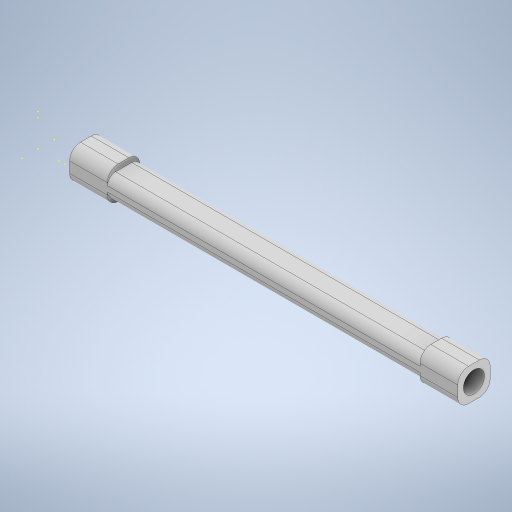
# Autodesk Inventor part: Part4
Saved by Autodesk Inventor 2024 (Build 280153000, 153)
## iProperties
Created: 2023-10-06
Part Number: Part4
Material: Generic
Document SubType Name: Modeling
Designer: kubad
Density: 1 g/cm^3
Appearance: Default
Author: kubad
## iProperties of the stored document Part3_3DPrint.ipt
Created: 2023-10-06
Part Number: Part3_3DPrint
Material: Generic
Document SubType Name: Modeling
Designer: kubad
Density: 1 g/cm^3
Appearance: Default
Author: kubad
Autodesk Inventor part; units mm, degrees
ref_plane "YZ Plane" through (0, 0, 0) normal (1, 0, 0) x (0, 1, 0)
ref_plane "XZ Plane" through (0, 0, 0) normal (0, 1, 0) x (-1, 0, 0)
ref_plane "XY Plane" through (0, 0, 0) normal (0, 0, 1) x (1, 0, 0)
sketch "Sketch1" plane through (0, 0, 0) normal (0, 1, 0) x (-1, 0, 0)
  point P0 (0, 0)
sketch "Sketch2" plane through (0, 0, 0) normal (0, 1, 0) x (-1, 0, 0)
  circle A0 centre (0, 0) radius 3.85
  dimension "d0" = 7.7
  constraints: 1 centre point, 1 coincident
  measures "d0" diameter of A0
extrude "Extrusion1" add sketch "Sketch2" along normal blind 6
sketch "Sketch3" plane through (0, 6, 0) normal (0, 1, 0) x (1, 0, 0)
  circle A0 centre (0, 0) radius 1
  dimension "d3" = 2
  constraints: 1 centre point, 1 coincident
  measures "d3" diameter of A0
extrude "Extrusion2" cut sketch "Sketch3" against normal through all
sketch "Sketch4" plane through (0, 0, 0) normal (0, -1, 0) x (1, 0, 0)
  circle A0 centre (0, 0) radius 3.85 projected
  line L0 (0, 3.85) -> (3.85, 3.85)
  line L1 (3.85, 3.85) -> (3.85, -3.85)
  line L2 (3.85, -3.85) -> (0, -3.85)
  line L3 (3.85, 3.85) -> (4.85, 3.85)
  line L4 (4.85, 3.85) -> (4.85, -3.85)
  line L5 (4.85, -3.85) -> (3.85, -3.85)
  line L6 (3.85, -3.85) -> (3.85, 3.85)
  line L7 (4.85, 3.85) -> (4.85, 3)
  line L8 (4.85, -3.85) -> (4.85, -3)
  line L9 (4.85, 3) -> (3.85, 3)
  line L10 (3.85, 3) -> (3.85, -3)
  line L11 (3.85, -3) -> (4.85, -3)
  line L12 (4.85, -3) -> (4.85, 3)
  point P0 (3.85, -3)
  dimension "d6" = 1
  dimension "d7" = 0.85
  dimension "d8" = 0.85
  constraints: 26 end point, 5 parallel, 4 point on line, 3 horizontal, 3 perpendicular, 1 vertical alignment, 1 other
  measures "d6" distance of L4.end L5.end
  measures "d7" distance of L3.end L7.end
  measures "d8" distance of L4.end L8.end
extrude "Extrusion3" add sketch "Sketch4" against normal blind 6 contours L1 L9 L4 L11
sketch "Sketch5" plane through (4.85, 0, 3) normal (1, 0, 0) x (0, 0, -1)
  line L0 (6.85, 0) -> (-0.85, 0) projected
  line L1 (6, 0) -> (6, 6) projected
  line L2 (0.0003, 0) -> (6, 0)
  line L3 (6, 0) -> (6, 1)
  line L4 (6, 1) -> (0.0003, 1)
  line L5 (0.0003, 1) -> (0.0003, 0)
  line L6 (6.85, 6) -> (-0.85, 6) projected
  line L7 (0.0003, 6) -> (6, 6)
  line L8 (6, 6) -> (6, 5)
  line L9 (6, 5) -> (0.0003, 5)
  line L10 (0.0003, 5) -> (0.0003, 6)
  point P0 (3, 0)
  point P1 (3, 6)
  dimension "d11" = 1
  dimension "d12" = 1
  constraints: 16 end point, 4 parallel, 4 point on line, 2 horizontal, 2 perpendicular
  measures "d11" distance of L3.end L2.end
  measures "d12" distance of L7.end L8.end
extrude "Extrusion4" cut sketch "Sketch5" against normal blind 1 contours L9 L10 L6 L1
extrude "Extrusion5" cut sketch "Sketch5" against normal blind 1 contours L0 L5 L4 L1
sketch "Sketch6" plane through (4.85, 5, 2.9997) normal (0, 0, -1) x (-1, 0, 0)
  line L0 (0, 0) -> (1, 0) projected
  line L1 (0, -5) -> (0, 1) projected
  line L2 (1, 0) -> (0, 0)
  line L3 (0, 0) -> (0, 1)
  line L4 (0, 1) -> (1, 1)
  line L5 (1, 1) -> (1, 0)
  line L6 (1, -5) -> (0, -5)
  line L7 (0, -5) -> (0, -3.9916)
  line L8 (0, -3.9916) -> (1, -3.9916)
  line L9 (1, -3.9916) -> (1, -5)
  point P0 (4.85, -5)
  constraints: 16 end point, 4 parallel, 2 horizontal, 2 perpendicular, 2 point on line
extrude "Extrusion6" cut sketch "Sketch6" against normal through all contours L1 L4 L5 L0
extrude "Extrusion7" cut sketch "Sketch6" against normal through all contours L1 L8 L9 L6
sketch "Sketch7" plane through (4.85, 5, 3) normal (1, 0, 0) x (0, 0, -1)
  line L0 (0, 0) -> (3, 0) projected
  line L1 (6, -4) -> (6, 0) projected
  line L2 (0, 0) -> (6, 0)
  line L3 (6, 0) -> (6, -4)
  line L4 (6, -4) -> (0, -4)
  line L5 (0, -4) -> (0, 0)
  point P0 (3, -5)
  constraints: 8 end point, 2 parallel, 1 horizontal, 1 perpendicular
extrude "Extrusion8" add sketch "Sketch7" along normal blind 71
sketch "Sketch8" plane through (3.85, 1, -3) normal (0, 0, -1) x (-1, 0, 0)
  point P0 (3.85, -1)
sketch "Sketch9" plane through (3.85, 5, 0) normal (0, 1, 0) x (1, 0, 0)
  line L0 (72, 3) -> (72, -3) projected
  line L1 (72, 0) -> (75.85, 0)
  circle A0 centre (75.85, 0) radius 3.85
  point P0 (-3.85, 0)
  dimension "d23" = 3.85
  constraints: 2 end point, 1 coincident, 1 horizontal, 1 horizontal alignment, 1 midpoint, 2 other
  measures "d23" distance of L1.start L1.end
extrude "Extrusion9" add sketch "Sketch9" along normal blind 1
extrude "Extrusion10" add sketch "Sketch9" against normal blind 5
sketch "Sketch10" plane through (79.7, 6, 0) normal (0, 1, 0) x (1, 0, 0)
  circle A0 centre (0, 0) radius 1.85
  point P0 (-79.7, 0)
  dimension "d28" = 3.7
  constraints: 1 centre point
  measures "d28" diameter of A0
extrude "Extrusion11" cut sketch "Sketch10" against normal through all
sketch "Sketch11" plane through (3.85, 5, 0) normal (-1, 0, 0) x (0, 0, 1)
  point P0 (0, -5)
sketch "Sketch12" plane through (3.85, 5, -3) normal (-1, 0, 0) x (0, 0, 1)
  line L0 (0, 0) -> (3, 0) projected
  line L1 (6, 0) -> (6, -4) projected
  line L2 (0, 0) -> (6, 0)
  line L3 (6, 0) -> (6, -4)
  line L4 (6, -4) -> (0, -4)
  line L5 (0, -4) -> (0, 0)
  point P0 (3, -5)
  constraints: 8 end point, 2 parallel, 1 horizontal, 1 perpendicular
extrude "Extrusion12" add sketch "Sketch12" along normal blind 2
sketch "Sketch13" plane through (75.85, 5, 3) normal (1, 0, 0) x (0, 0, -1)
  line L0 (3, 0) -> (0, 0) projected
  line L1 (3, -4) -> (6, -4) projected
  line L2 (0, 0) -> (6, 0)
  line L3 (6, 0) -> (6, -4)
  line L4 (6, -4) -> (0, -4)
  line L5 (0, -4) -> (0, 0)
  point P0 (3, -5)
  constraints: 8 end point, 2 parallel, 1 horizontal, 1 perpendicular
extrude "Extrusion13" add sketch "Sketch13" along normal blind 1.6
fillet "Fillet1" radius 1.5 1 edges at (39.85, 5, 3)
fillet "Fillet2" radius 1.5 1 edges at (39.85, 5, -3)
fillet "Fillet3" radius 1.5 1 edges at (39.85, 1, -3)
fillet "Fillet4" radius 1.5 1 edges at (41.0685, 1, 3)
sketch "Sketch14" plane through (3.5458, 5, 1.5) normal (0, 1, 0) x (1, 0, 0)
  point P0 (-3.5458, 1.5)
sketch "Sketch15" plane through (3.5458, 5, 1.5) normal (0, 1, 0) x (1, 0, 0)
  line L0 (0.4177, 2.9988) -> (2.9717, 2.9988) construction
  line L1 (2.9717, 2.9988) -> (2.9717, -0.0492) construction
  line L2 (2.9717, -0.0492) -> (0.4177, -0.0492) construction
  line L3 (0.4177, -0.0492) -> (0.4177, 2.9988) construction
  line L4 (0.398, -0.0492) -> (1.4255, 2.9988)
  line L5 (1.4255, 2.9988) -> (1.9244, 2.9988)
  line L6 (1.9244, 2.9988) -> (2.952, -0.0492)
  line L7 (2.952, -0.0492) -> (2.5247, -0.0492)
  line L8 (2.5247, -0.0492) -> (2.248, 0.803)
  line L9 (2.248, 0.803) -> (1.0846, 0.803)
  line L10 (1.0846, 0.803) -> (0.808, -0.0492)
  line L11 (0.808, -0.0492) -> (0.398, -0.0492)
  line L12 (2.1369, 1.1488) -> (1.6651, 2.5839)
  line L13 (1.6651, 2.5839) -> (1.1958, 1.1488)
  line L14 (1.1958, 1.1488) -> (2.1369, 1.1488)
  point P0 (-3.5458, 1.5)
  constraints: 2 other
extrude "Extrusion14" add sketch "Sketch15" along normal blind 0.2
sketch "Sketch16" plane through (3.5458, 5, -1.5) normal (0, 1, 0) x (1, 0, 0)
  line L0 (69.8363, -0.0038) -> (72.3064, -0.0038) construction
  line L1 (72.3064, -0.0038) -> (72.3064, -3.0518) construction
  line L2 (72.3064, -3.0518) -> (69.8363, -3.0518) construction
  line L3 (69.8363, -3.0518) -> (69.8363, -0.0038) construction
  spline S0 degree 2 poles (72.2125, -2.1157) (72.2125, -2.3429) (72.0396, -2.6912) (71.8963, -2.8048) knots 0 0 0 1 2 2 2
  spline S1 degree 2 poles (71.8963, -2.8048) (71.7234, -2.9382) (71.3307, -3.0518) (71.0195, -3.0518) knots 0 0 0 1 2 2 2
  line L4 (71.0195, -3.0518) -> (70.1451, -3.0518)
  line L5 (70.1451, -3.0518) -> (70.1451, -0.0038)
  line L6 (70.1451, -0.0038) -> (70.9528, -0.0038)
  spline S2 degree 2 poles (70.9528, -0.0038) (71.2788, -0.0038) (71.6049, -0.0458) (71.7531, -0.1273) knots 0 0 0 1 2 2 2
  spline S3 degree 2 poles (71.7531, -0.1273) (71.9186, -0.2138) (72.0692, -0.4978) (72.0692, -0.6905) knots 0 0 0 1 2 2 2
  spline S4 degree 2 poles (72.0692, -0.6905) (72.0692, -0.9054) (71.842, -1.2462) (71.6419, -1.3426) knots 0 0 0 1 2 2 2
  line L7 (71.6419, -1.3426) -> (71.6419, -1.3574)
  spline S5 degree 2 poles (71.6419, -1.3574) (71.9136, -1.4315) (72.2125, -1.8242) (72.2125, -2.1157) knots 0 0 0 1 2 2 2
  spline S6 degree 2 poles (71.7901, -2.133) (71.7901, -1.9601) (71.6913, -1.7378) (71.5431, -1.6587) knots 0 0 0 1 2 2 2
  spline S7 degree 2 poles (71.5431, -1.6587) (71.4468, -1.6093) (71.2195, -1.5797) (71.0096, -1.5797) knots 0 0 0 1 2 2 2
  line L8 (71.0096, -1.5797) -> (70.5502, -1.5797)
  line L9 (70.5502, -1.5797) -> (70.5502, -2.706)
  line L10 (70.5502, -2.706) -> (70.8787, -2.706)
  spline S8 degree 2 poles (70.8787, -2.706) (71.1454, -2.706) (71.4517, -2.6566) (71.5703, -2.5776) knots 0 0 0 1 2 2 2
  spline S9 degree 2 poles (71.5703, -2.5776) (71.6839, -2.4961) (71.7901, -2.2935) (71.7901, -2.133) knots 0 0 0 1 2 2 2
  spline S10 degree 2 poles (71.6469, -0.7473) (71.6469, -0.6386) (71.5728, -0.4756) (71.4912, -0.4287) knots 0 0 0 1 2 2 2
  spline S11 degree 2 poles (71.4912, -0.4287) (71.3924, -0.3743) (71.1529, -0.3496) (70.938, -0.3496) knots 0 0 0 1 2 2 2
  line L11 (70.938, -0.3496) -> (70.5502, -0.3496)
  line L12 (70.5502, -0.3496) -> (70.5502, -1.2413)
  line L13 (70.5502, -1.2413) -> (71.0096, -1.2413)
  spline S12 degree 2 poles (71.0096, -1.2413) (71.1998, -1.2413) (71.3801, -1.2018) (71.4764, -1.14) knots 0 0 0 1 2 2 2
  spline S13 degree 2 poles (71.4764, -1.14) (71.5703, -1.0807) (71.6469, -0.8905) (71.6469, -0.7473) knots 0 0 0 1 2 2 2
  point P0 (-3.5458, -1.5)
  constraints: 2 other
extrude "Extrusion15" add sketch "Sketch16" along normal blind 0.2
sketch "Sketch17" plane through (3.5458, 5, -1.5) normal (0, 1, 0) x (1, 0, 0)
  line L0 (0.4145, -1.5) -> (36.4145, -1.5)
  line L1 (30.4487, 0.0859) -> (55.6072, 0.0859) construction
  line L2 (55.6072, 0.0859) -> (55.6072, -2.5363) construction
  line L3 (55.6072, -2.5363) -> (30.4487, -2.5363) construction
  line L4 (30.4487, -2.5363) -> (30.4487, 0.0859) construction
  line L5 (32.5853, -0.4353) -> (31.2663, -3.0264)
  line L6 (31.2663, -3.0264) -> (30.8316, -3.0264)
  line L7 (30.8316, -3.0264) -> (32.2247, -0.3365)
  line L8 (32.2247, -0.3365) -> (30.6513, -0.3365)
  line L9 (30.6513, -0.3365) -> (30.6513, 0.0216)
  line L10 (30.6513, 0.0216) -> (32.5853, 0.0216)
  line L11 (32.5853, 0.0216) -> (32.5853, -0.4353)
  line L12 (34.838, -3.0264) -> (32.9583, -3.0264)
  line L13 (32.9583, -3.0264) -> (32.9583, -2.5941)
  spline S0 degree 2 poles (32.9583, -2.5941) (33.1608, -2.4039) (33.5214, -2.0507) (33.6943, -1.8605) knots 0 0 0 1 2 2 2
  spline S1 degree 2 poles (33.6943, -1.8605) (34.0426, -1.4777) (34.297, -1.0182) (34.297, -0.7737) knots 0 0 0 1 2 2 2
  spline S2 degree 2 poles (34.297, -0.7737) (34.297, -0.6453) (34.218, -0.4526) (34.1464, -0.3909) knots 0 0 0 1 2 2 2
  spline S3 degree 2 poles (34.1464, -0.3909) (34.0747, -0.3291) (33.887, -0.2674) (33.7734, -0.2674) knots 0 0 0 1 2 2 2
  spline S4 degree 2 poles (33.7734, -0.2674) (33.6647, -0.2674) (33.4424, -0.3217) (33.3411, -0.3637) knots 0 0 0 1 2 2 2
  spline S5 degree 2 poles (33.3411, -0.3637) (33.2547, -0.3983) (33.0941, -0.4971) (33.0447, -0.5317) knots 0 0 0 1 2 2 2
  line L14 (33.0447, -0.5317) -> (33.0225, -0.5317)
  line L15 (33.0225, -0.5317) -> (33.0225, -0.0969)
  spline S6 degree 2 poles (33.0225, -0.0969) (33.1485, -0.0352) (33.6005, 0.0859) (33.803, 0.0859) knots 0 0 0 1 2 2 2
  spline S7 degree 2 poles (33.803, 0.0859) (34.2303, 0.0859) (34.712, -0.3662) (34.712, -0.7515) knots 0 0 0 1 2 2 2
  spline S8 degree 2 poles (34.712, -0.7515) (34.712, -0.9318) (34.628, -1.2331) (34.5539, -1.3616) knots 0 0 0 1 2 2 2
  spline S9 degree 2 poles (34.5539, -1.3616) (34.4798, -1.495) (34.2649, -1.7568) (34.1464, -1.8828) knots 0 0 0 1 2 2 2
  spline S10 degree 2 poles (34.1464, -1.8828) (33.9537, -2.0927) (33.4819, -2.5422) (33.3411, -2.6732) knots 0 0 0 1 2 2 2
  line L16 (33.3411, -2.6732) -> (34.838, -2.6732)
  line L17 (34.838, -2.6732) -> (34.838, -3.0264)
  line L18 (37.8958, -3.0264) -> (37.8958, -1.7024)
  spline S11 degree 2 poles (37.8958, -1.7024) (37.8958, -1.5444) (37.8711, -1.2751) (37.8316, -1.201) knots 0 0 0 1 2 2 2
  spline S12 degree 2 poles (37.8316, -1.201) (37.7921, -1.1195) (37.6414, -1.0405) (37.5105, -1.0405) knots 0 0 0 1 2 2 2
  spline S13 degree 2 poles (37.5105, -1.0405) (37.392, -1.0405) (37.1203, -1.1862) (36.977, -1.3245) knots 0 0 0 1 2 2 2
  spline S14 degree 2 poles (36.977, -1.3245) (36.9795, -1.3591) (36.9844, -1.4554) (36.9844, -1.5197) knots 0 0 0 1 2 2 2
  line L19 (36.9844, -1.5197) -> (36.9844, -3.0264)
  line L20 (36.9844, -3.0264) -> (36.5991, -3.0264)
  line L21 (36.5991, -3.0264) -> (36.5991, -1.7024)
  spline S15 degree 2 poles (36.5991, -1.7024) (36.5991, -1.5444) (36.5744, -1.2751) (36.5349, -1.201) knots 0 0 0 1 2 2 2
  spline S16 degree 2 poles (36.5349, -1.201) (36.4953, -1.1195) (36.3447, -1.0405) (36.2138, -1.0405) knots 0 0 0 1 2 2 2
  spline S17 degree 2 poles (36.2138, -1.0405) (36.0903, -1.0405) (35.8161, -1.1961) (35.6876, -1.3171) knots 0 0 0 1 2 2 2
  line L22 (35.6876, -1.3171) -> (35.6876, -3.0264)
  line L23 (35.6876, -3.0264) -> (35.3023, -3.0264)
  line L24 (35.3023, -3.0264) -> (35.3023, -0.7391)
  line L25 (35.3023, -0.7391) -> (35.6876, -0.7391)
  line L26 (35.6876, -0.7391) -> (35.6876, -0.9911)
  spline S18 degree 2 poles (35.6876, -0.9911) (35.8383, -0.8404) (36.1347, -0.6749) (36.3126, -0.6749) knots 0 0 0 1 2 2 2
  spline S19 degree 2 poles (36.3126, -0.6749) (36.5151, -0.6749) (36.8288, -0.8602) (36.9103, -1.0701) knots 0 0 0 1 2 2 2
  spline S20 degree 2 poles (36.9103, -1.0701) (37.0857, -0.875) (37.4167, -0.6749) (37.6093, -0.6749) knots 0 0 0 1 2 2 2
  spline S21 degree 2 poles (37.6093, -0.6749) (37.7575, -0.6749) (37.9996, -0.7663) (38.0885, -0.87) knots 0 0 0 1 2 2 2
  spline S22 degree 2 poles (38.0885, -0.87) (38.1799, -0.9738) (38.2812, -1.285) (38.2812, -1.5197) knots 0 0 0 1 2 2 2
  line L27 (38.2812, -1.5197) -> (38.2812, -3.0264)
  line L28 (38.2812, -3.0264) -> (37.8958, -3.0264)
  line L29 (41.4156, -3.0264) -> (41.4156, -1.7024)
  spline S23 degree 2 poles (41.4156, -1.7024) (41.4156, -1.5444) (41.3909, -1.2751) (41.3514, -1.201) knots 0 0 0 1 2 2 2
  spline S24 degree 2 poles (41.3514, -1.201) (41.3119, -1.1195) (41.1612, -1.0405) (41.0303, -1.0405) knots 0 0 0 1 2 2 2
  spline S25 degree 2 poles (41.0303, -1.0405) (40.9117, -1.0405) (40.64, -1.1862) (40.4968, -1.3245) knots 0 0 0 1 2 2 2
  spline S26 degree 2 poles (40.4968, -1.3245) (40.4992, -1.3591) (40.5042, -1.4554) (40.5042, -1.5197) knots 0 0 0 1 2 2 2
  line L30 (40.5042, -1.5197) -> (40.5042, -3.0264)
  line L31 (40.5042, -3.0264) -> (40.1189, -3.0264)
  line L32 (40.1189, -3.0264) -> (40.1189, -1.7024)
  spline S27 degree 2 poles (40.1189, -1.7024) (40.1189, -1.5444) (40.0942, -1.2751) (40.0546, -1.201) knots 0 0 0 1 2 2 2
  spline S28 degree 2 poles (40.0546, -1.201) (40.0151, -1.1195) (39.8644, -1.0405) (39.7335, -1.0405) knots 0 0 0 1 2 2 2
  spline S29 degree 2 poles (39.7335, -1.0405) (39.61, -1.0405) (39.3359, -1.1961) (39.2074, -1.3171) knots 0 0 0 1 2 2 2
  line L33 (39.2074, -1.3171) -> (39.2074, -3.0264)
  line L34 (39.2074, -3.0264) -> (38.8221, -3.0264)
  line L35 (38.8221, -3.0264) -> (38.8221, -0.7391)
  line L36 (38.8221, -0.7391) -> (39.2074, -0.7391)
  line L37 (39.2074, -0.7391) -> (39.2074, -0.9911)
  spline S30 degree 2 poles (39.2074, -0.9911) (39.3581, -0.8404) (39.6545, -0.6749) (39.8323, -0.6749) knots 0 0 0 1 2 2 2
  spline S31 degree 2 poles (39.8323, -0.6749) (40.0349, -0.6749) (40.3486, -0.8602) (40.4301, -1.0701) knots 0 0 0 1 2 2 2
  spline S32 degree 2 poles (40.4301, -1.0701) (40.6054, -0.875) (40.9364, -0.6749) (41.1291, -0.6749) knots 0 0 0 1 2 2 2
  spline S33 degree 2 poles (41.1291, -0.6749) (41.2773, -0.6749) (41.5194, -0.7663) (41.6083, -0.87) knots 0 0 0 1 2 2 2
  spline S34 degree 2 poles (41.6083, -0.87) (41.6997, -0.9738) (41.8009, -1.285) (41.8009, -1.5197) knots 0 0 0 1 2 2 2
  line L38 (41.8009, -1.5197) -> (41.8009, -3.0264)
  line L39 (41.8009, -3.0264) -> (41.4156, -3.0264)
  point P0 (-3.5458, -1.5)
  dimension "d43" = 36
  constraints: 2 end point, 1 horizontal, 2 other
  measures "d43" distance of L0.start L0.end
extrude "Extrusion16" add sketch "Sketch17" along normal blind 0.2
sketch "Sketch18" plane through (3.5458, 5.2, -1.5) normal (0, 1, 0) x (1, 0, 0)
  line L0 (29.8828, 2.0952) -> (43.3392, 2.0952)
  line L1 (43.3392, 2.0952) -> (43.3392, -5.5663)
  line L2 (43.3392, -5.5663) -> (29.8828, -5.5663)
  line L3 (29.8828, -5.5663) -> (29.8828, 2.0952)
  point P0 (-3.5458, -1.5)
  constraints: 8 end point, 2 parallel, 1 horizontal, 1 perpendicular
extrude "Extrusion17" cut sketch "Sketch18" against normal blind 0.2
sketch "Sketch19" plane through (3.5458, 5.2, 1.5) normal (0, 1, 0) x (1, 0, 0)
  line L0 (0.3624, -0.1736) -> (3.3783, -0.1736)
  line L1 (3.3783, -0.1736) -> (3.3783, 3.2897)
  line L2 (3.3783, 3.2897) -> (0.3624, 3.2897)
  line L3 (0.3624, 3.2897) -> (0.3624, -0.1736)
  line L4 (72.2697, -0.5369) -> (69.8008, -0.5369)
  line L5 (69.8008, -0.5369) -> (69.8008, 3.7021)
  line L6 (69.8008, 3.7021) -> (72.2697, 3.7021)
  line L7 (72.2697, 3.7021) -> (72.2697, -0.5369)
  point P0 (-3.5458, 1.5)
  constraints: 16 end point, 4 parallel, 2 horizontal, 2 perpendicular
extrude "Extrusion18" cut sketch "Sketch19" against normal blind 0.2 contours L3 L2 L1 L0
extrude "Extrusion19" cut sketch "Sketch19" against normal blind 0.2 contours L4 L5 L6 L7
sketch "Sketch20" plane through (79.7, 0, 0) normal (0, -1, 0) x (1, 0, 0)
  point P0 (-79.7, 0)
sketch "Sketch21" plane through (79.7, 6, 0) normal (0, 1, 0) x (1, 0, 0)
  circle A0 centre (0, 0) radius 1.95
  point P0 (-79.7, 0)
  dimension "d52" = 3.9
  constraints: 1 centre point
  measures "d52" diameter of A0
extrude "Extrusion20" cut sketch "Sketch21" against normal through all
sketch "Sketch22" plane through (0, 6, 0) normal (0, 1, 0) x (1, 0, 0)
  line L0 (0, 0) -> (0, -3.85)
  circle A0 centre (0, 0) radius 3.85 projected
  line L1 (0, -3.85) -> (3.85, -3.85)
  line L2 (3.85, -3.85) -> (-3.85, -3.85)
  line L3 (-3.85, -3.85) -> (-3.85, 3.85)
  line L4 (-3.85, 3.85) -> (3.85, 3.85)
  line L5 (3.85, 3.85) -> (3.85, -3.85)
  constraints: 12 end point, 3 horizontal, 2 parallel, 1 perpendicular, 1 vertical, 1 vertical alignment, 1 other
extrude "Extrusion21" cut sketch "Sketch22" against normal through all contours A0
sketch "Sketch23" plane through (79.7, 5, 0) normal (0, 1, 0) x (1, 0, 0)
  arc A0 (-76.1542, -1.5) -> (-76.1542, 1.5) centre (-79.7, 0) ccw projected
  line L0 (-75.85, 0) -> (-77.9753, 0)
  line L1 (-77.9753, 0) -> (-77.9753, 3.5992)
  line L2 (-77.9753, 3.5992) -> (-75.85, 3.5992)
  line L3 (-75.85, 3.5992) -> (-75.85, 0)
  line L4 (-75.85, 0) -> (-77.9753, 0)
  line L5 (-77.9753, 0) -> (-77.9753, -3.4561)
  line L6 (-77.9753, -3.4561) -> (-75.85, -3.4561)
  line L7 (-75.85, -3.4561) -> (-75.85, 0)
  line L8 (-75.85, -3.4561) -> (-65.85, -3.4561)
  line L9 (-65.85, -3.4561) -> (-65.85, 3.5992)
  line L10 (-65.85, 3.5992) -> (-75.85, 3.5992)
  line L11 (-75.85, 3.5992) -> (-75.85, -3.4561)
  dimension "d57" = 10
  constraints: 24 end point, 6 parallel, 3 horizontal, 3 perpendicular, 2 point on line, 1 point on circle
  measures "d57" distance of L10.end L9.end
extrude "Extrusion22" cut sketch "Sketch23" against normal through all contours L3 L10 L9 L8 L7
extrude "Extrusion23" cut sketch "Sketch23" against normal through all contours L7 L6 L5 L0
extrude "Extrusion24" cut sketch "Sketch23" against normal through all contours L0 L1 L2 L3
sketch "Sketch24" plane through (13.85, 5, -1.5) normal (-1, 0, 0) x (0, 0, 1)
  line L0 (-2.9013, -5) -> (5.7799, -5)
  line L1 (5.7799, -5) -> (5.7799, 1.344)
  line L2 (5.7799, 1.344) -> (-2.9013, 1.344)
  line L3 (-2.9013, 1.344) -> (-2.9013, -5)
  point P0 (1.5, -5)
  constraints: 8 end point, 2 parallel, 1 horizontal, 1 perpendicular
extrude "Extrusion25" cut sketch "Sketch24" against normal blind 6.142
sketch "Sketch25" plane through (19.992, 5, -1.5) normal (-1, 0, 0) x (0, 0, 1)
  line L0 (-1.5, 0) -> (4.5, 0)
  line L1 (4.5, 0) -> (4.5, -4)
  line L2 (4.5, -4) -> (-1.5, -4)
  line L3 (-1.5, -4) -> (-1.5, 0)
  point P0 (1.5, -5)
  dimension "d66" = 6
  dimension "d67" = 4
  constraints: 8 end point, 2 parallel, 1 horizontal, 1 perpendicular
  measures "d66" distance of L1.end L2.end
  measures "d67" distance of L0.end L1.end
extrude "Extrusion26" add sketch "Sketch25" along normal blind 6.133
sketch "Sketch26" plane through (79.7, 6, 0) normal (0, 1, 0) x (1, 0, 0)
  line L0 (-65.841, -3) -> (-65.841, 3) projected
  line L1 (-65.841, 0) -> (-69.691, 0)
  circle A0 centre (-69.691, 0) radius 3.85
  point P0 (-79.7, 0)
  dimension "d70" = 3.85
  constraints: 2 end point, 1 centre point, 1 coincident, 1 horizontal, 1 midpoint, 1 tangent
  measures "d70" distance of L1.start L1.end
extrude "Extrusion27" add sketch "Sketch26" against normal blind 6
sketch "Sketch27" plane through (13.859, 5, -1.5) normal (-1, 0, 0) x (0, 0, 1)
  point P0 (1.5, -5)
sketch "Sketch28" plane through (13.859, 5, -1.5) normal (-1, 0, 0) x (0, 0, 1)
  line L0 (-1.5, 0) -> (-1.5, -4) projected
  line L1 (4.5, 0) -> (3, 0) projected
  line L2 (-1.5, -4) -> (4.5, -4)
  line L3 (4.5, -4) -> (4.5, 0)
  line L4 (4.5, 0) -> (-1.5, 0)
  line L5 (-1.5, 0) -> (-1.5, -4)
  point P0 (1.5, -5)
  constraints: 8 end point, 2 parallel, 1 horizontal, 1 perpendicular
extrude "Extrusion28" add sketch "Sketch28" along normal blind 5
sketch "Sketch29" plane through (19.992, 3.5, 3) normal (0, 0, 1) x (1, 0, 0)
  point P0 (-19.992, -3.5)
sketch "Sketch30" plane through (79.7, 5, 0) normal (0, 1, 0) x (1, 0, 0)
  point P0 (-79.7, 0)
sketch "Sketch31" plane through (19.992, 5, -1.5) normal (1, 0, 0) x (0, 0, -1)
  arc A0 (-3, 0) -> (-4.5, -1.5) centre (-3, -1.5) ccw projected
  circle A1 centre (-3, -1.5) radius 1.5
  circle A2 centre (-3, -1.5) radius 1.5
  arc A3 (-4.5, -2.5) -> (-3, -4) centre (-3, -2.5) ccw projected
  circle A4 centre (-3, -2.5) radius 1.5
  arc A5 (0, -4) -> (1.5, -2.5) centre (0, -2.5) ccw projected
  circle A6 centre (0, -2.5) radius 1.5
  arc A7 (1.5, -1.5) -> (0, 0) centre (0, -1.5) ccw projected
  circle A8 centre (0, -1.5) radius 1.5
  line L0 (-4.5, -1.5) -> (-4.5, 0) projected
  line L1 (-4.5, 0) -> (-3, 0)
  line L2 (-3, 0) -> (-3, -1.5)
  line L3 (-3, -1.5) -> (-4.5, -1.5)
  line L4 (-4.5, -1.5) -> (-4.5, 0)
  line L5 (0, 0) -> (1.5, 0)
  line L6 (1.5, 0) -> (1.5, -1.5)
  line L7 (1.5, -1.5) -> (0, -1.5)
  line L8 (0, -1.5) -> (0, 0)
  line L9 (-3, -4) -> (-4.5, -4)
  line L10 (-4.5, -4) -> (-4.5, -2.5)
  line L11 (-4.5, -2.5) -> (-3, -2.5)
  line L12 (-3, -2.5) -> (-3, -4)
  line L13 (0, -4) -> (1.5, -4)
  line L14 (1.5, -4) -> (1.5, -2.5)
  line L15 (1.5, -2.5) -> (0, -2.5)
  line L16 (0, -2.5) -> (0, -4)
  point P0 (-1.5, -5)
  constraints: 32 end point, 8 parallel, 5 coincident, 4 horizontal, 4 perpendicular, 3 centre point, 1 horizontal alignment, 1 point on line, 1 vertical alignment, 5 other
extrude "Extrusion29" cut sketch "Sketch31" against normal blind 10 contours A0 L0 L1
extrude "Extrusion30" cut sketch "Sketch31" against normal blind 10 contours A3 L9 L10
extrude "Extrusion31" cut sketch "Sketch31" against normal blind 10 contours A5 L14 L13
extrude "Extrusion32" cut sketch "Sketch31" against normal blind 10 contours L5 L6 A7
sketch "Sketch32" plane through (79.7, 6, 0) normal (0, 1, 0) x (1, 0, 0)
  point P0 (-79.7, 0)
sketch "Sketch33" plane through (10.009, 6, 0) normal (0, 1, 0) x (1, 0, 0)
  circle A0 centre (0, 0) radius 3.85
  point P0 (-10.009, 0)
  constraints: 1 centre point
extrude "Extrusion33" add sketch "Sketch33" against normal blind 6
sketch "Sketch34" plane through (10.009, 6, 0) normal (0, 1, 0) x (1, 0, 0)
  circle A0 centre (0, 0) radius 1.925
  point P0 (-10.009, 0)
  dimension "d85" = 3.85
  constraints: 1 centre point
  measures "d85" diameter of A0
extrude "Extrusion34" cut sketch "Sketch34" against normal blind 6
sketch "Sketch35" plane through (10.009, 6, 0) normal (0, 1, 0) x (1, 0, 0)
  point P0 (-10.009, 0)
sketch "Sketch36" plane through (79.7, 6, 0) normal (0, 1, 0) x (1, 0, 0)
  point P0 (-79.7, 0)
sketch "Sketch37" plane through (79.7, 6, 0) normal (0, 1, 0) x (1, 0, 0)
  point P0 (-79.7, 0)
sketch "Sketch38" plane through (10.009, 6, 0) normal (0, 1, 0) x (1, 0, 0)
  circle A0 centre (0, 0) radius 1.95
  point P0 (-10.009, 0)
  dimension "d89" = 3.9
  constraints: 1 centre point
  measures "d89" diameter of A0
extrude "Extrusion35" cut sketch "Sketch38" against normal blind 6
sketch "Sketch39" plane through (79.7, 6, 0) normal (0, 1, 0) x (1, 0, 0)
  point P0 (-79.7, 0)
sketch "Sketch40" plane through (79.7, 6, 0) normal (0, 1, 0) x (1, 0, 0)
  point P0 (-79.7, 0)
sketch "Sketch41" plane through (79.7, 6, 0) normal (0, 1, 0) x (1, 0, 0)
  point P0 (-79.7, 0)
sketch "Sketch42" plane through (79.7, 6, 0) normal (0, 1, 0) x (1, 0, 0)
  circle A0 centre (0, 0) radius 3
  arc A1 (-66.1452, -1.5) -> (-66.1452, 1.5) centre (-69.691, 0) ccw projected
  circle A2 centre (-69.691, 0) radius 3
  point P0 (-79.7, 0)
  dimension "d92" = 6
  dimension "d93" = 6
  constraints: 2 centre point, 1 coincident
  measures "d92" diameter of A0
  measures "d93" diameter of A2
extrude "Extrusion36" cut sketch "Sketch42" against normal through all contours A0
extrude "Extrusion37" cut sketch "Sketch42" against normal through all contours A2
sketch "Sketch43" plane through (10.009, 0, 0) normal (0, -1, 0) x (1, 0, 0)
  circle A0 centre (0, 0) radius 3.85 projected
  line L0 (0, 3.85) -> (-5, 3.85)
  line L1 (-5, 3.85) -> (-5, -3.85)
  line L2 (-5, -3.85) -> (0, -3.85)
  line L3 (0, -3.85) -> (0, 3.85)
  line L4 (-5, 3.85) -> (-4.5, 3.85)
  line L5 (-4.5, 3.85) -> (-4.5, -3.85)
  line L6 (-4.5, -3.85) -> (-5, -3.85)
  line L7 (-5, -3.85) -> (-5, 3.85)
  point P0 (-10.009, 0)
  dimension "d98" = 5
  dimension "d99" = 0.5
  constraints: 16 end point, 4 parallel, 2 horizontal, 2 perpendicular, 1 point on line, 1 vertical alignment, 1 other
  measures "d98" distance of L2.end L1.end
  measures "d99" distance of L5.end L6.end
extrude "Extrusion38" add sketch "Sketch43" against normal blind 1 contours L5 L2 L1 L0
sketch "Sketch44" plane through (5.009, 0, -3.85) normal (-1, 0, 0) x (0, 0, 1)
  point P0 (3.85, 0)
sketch "Sketch45" plane through (5.009, 0, -3.85) normal (-1, 0, 0) x (0, 0, 1)
  line L0 (7.7, 1) -> (0, 1) projected
  line L1 (0, 0) -> (7.7, 0) projected
  line L2 (0, 1) -> (7.7, 1)
  line L3 (7.7, 1) -> (7.7, 0)
  line L4 (7.7, 0) -> (0, 0)
  line L5 (0, 0) -> (0, 1)
  point P0 (3.85, 0)
  constraints: 8 end point, 2 parallel, 1 horizontal, 1 perpendicular
extrude "Extrusion39" cut sketch "Sketch45" against normal through all
sketch "Sketch46" plane through (10.009, 6, 0) normal (0, 1, 0) x (1, 0, 0)
  circle A0 centre (0, 0) radius 3.85 projected
  line L0 (0, 3.85) -> (-5, 3.85)
  line L1 (-5, 3.85) -> (-5, -3.85)
  line L2 (-5, -3.85) -> (0, -3.85)
  line L3 (0, -3.85) -> (0, 3.85)
  line L4 (-5, 3.85) -> (-4.5, 3.85)
  line L5 (-4.5, 3.85) -> (-4.5, -3.85)
  line L6 (-4.5, -3.85) -> (-5, -3.85)
  line L7 (-5, -3.85) -> (-5, 3.85)
  point P0 (-10.009, 0)
  dimension "d104" = 5
  dimension "d105" = 0.5
  constraints: 16 end point, 4 parallel, 2 horizontal, 2 perpendicular, 1 point on line, 1 vertical alignment, 1 other
  measures "d104" distance of L2.end L1.end
  measures "d105" distance of L5.end L6.end
extrude "Extrusion40" add sketch "Sketch46" against normal blind 1 contours L5 L2 L1 L0
sketch "Sketch47" plane through (5.009, 6, -3.85) normal (-1, 0, 0) x (0, 0, 1)
  line L0 (0, 0) -> (0, -1) projected
  line L1 (0, -1) -> (7.7, -1) projected
  line L2 (0, 0) -> (7.7, 0)
  line L3 (7.7, 0) -> (7.7, -1)
  line L4 (7.7, -1) -> (0, -1)
  line L5 (0, -1) -> (0, 0)
  point P0 (3.85, -6)
  constraints: 8 end point, 2 parallel, 1 horizontal, 1 perpendicular
extrude "Extrusion41" cut sketch "Sketch47" against normal through all
sketch "Sketch48" plane through (12.422, 2.5, 3) normal (0, 0, 1) x (1, 0, 0)
  line L0 (1.1328, 2.5) -> (63.7322, 2.5) projected
  line L1 (1.1328, -1.5) -> (63.7322, -1.5) projected
  line L2 (63.7322, 2.5) -> (63.7322, -1.5)
  line L3 (63.7322, 2.5) -> (71.128, 2.5) projected
  line L4 (71.128, 2.5) -> (63.7322, -1.5)
  line L5 (63.7322, 2.5) -> (71.128, -1.5)
  line L6 (71.128, -1.5) -> (71.128, 2.5) projected
  circle A0 centre (67.4301, 0.5) radius 4.2041
  line L7 (67.4301, 0.5) -> (67.4301, -1.5)
  line L8 (64.278, -1.5) -> (70.278, -1.5) projected
  line L9 (70.278, 2.5) -> (70.278, -1.5) projected
  line L10 (71.128, 0.6263) -> (70.278, 0.6263)
  line L11 (63.7322, 0.5) -> (64.5822, 0.5)
  line L12 (64.5822, 2.5) -> (64.5822, -1.5)
  line L13 (70.278, 2.5) -> (70.278, -1.5)
  line L14 (64.5822, 2.5) -> (70.278, -1.5)
  line L15 (70.278, 2.5) -> (64.5822, -1.5)
  circle A1 centre (67.4301, 0.5) radius 3.48
  line L16 (63.7322, 2.5) -> (71.128, 2.5)
  point P0 (-12.422, -2.5)
  dimension "d110" = 4
  dimension "d111" = 0.85
  constraints: 22 end point, 6 point on line, 4 midpoint, 2 collinear, 2 perpendicular, 2 vertical, 1 horizontal, 6 other
  measures "d110" distance of L0.end L1.end
  measures "d111" distance of L11.start L11.end
extrude "Extrusion42" add sketch "Sketch48" against normal blind 6 contours A0 L3 A1
sketch "Sketch49" plane through (12.422, 2.5, 3) normal (0, 0, 1) x (1, 0, 0)
  line L0 (71.128, 2.5) -> (61.853, 2.5)
  line L1 (61.853, 2.5) -> (61.853, 6.3445)
  line L2 (61.853, 6.3445) -> (71.128, 6.3445)
  line L3 (71.128, 6.3445) -> (71.128, 2.5)
  point P0 (-12.422, -2.5)
  constraints: 8 end point, 2 parallel, 1 horizontal, 1 perpendicular
extrude "Extrusion43" cut sketch "Sketch49" against normal through all
sketch "Sketch50" plane through (79.7, 5, 0) normal (0, 1, 0) x (1, 0, 0)
  arc A0 (-3.5458, -1.5) -> (-3.5458, 1.5) centre (0, 0) ccw projected
  line L0 (0, -3.85) -> (3.85, -3.85)
  circle A1 centre (0, 0) radius 3.85
  line L1 (0, 3.85) -> (-3.85, 3.85)
  line L2 (-3.85, 3.85) -> (3.85, 3.85)
  line L3 (3.85, 3.85) -> (3.85, -3.85)
  line L4 (3.85, -3.85) -> (-3.85, -3.85)
  line L5 (-3.85, -3.85) -> (-3.85, 3.85)
  circle A2 centre (-69.691, 0) radius 3 projected
  arc A3 (-66.1452, 1.5) -> (-66.1452, -1.5) centre (-69.691, 0) ccw projected
  circle A4 centre (-69.691, 0) radius 3.85
  line L6 (-69.691, 3.85) -> (-73.541, 3.85)
  line L7 (-73.541, 3.85) -> (-65.841, 3.85)
  line L8 (-65.841, 3.85) -> (-65.841, -3.85)
  line L9 (-65.841, -3.85) -> (-73.541, -3.85)
  line L10 (-73.541, -3.85) -> (-73.541, 3.85)
  point P0 (-79.7, 0)
  point P1 (-3.85, 0)
  point P2 (-3.5458, -1.5)
  point P3 (-3.5458, 1.5)
  point P4 (-69.691, -3.85)
  point P5 (-65.841, 0)
  point P6 (-66.1452, -1.5)
  constraints: 22 end point, 6 horizontal, 4 parallel, 4 tangent, 3 point on circle, 2 coincident, 2 perpendicular, 1 centre point, 4 other
extrude "Extrusion44" cut sketch "Sketch50" against normal blind 10 contours A0 L4 L5 A1
extrude "Extrusion45" cut sketch "Sketch50" against normal blind 10 contours L5 L1 A0 A1
extrude "Extrusion46" cut sketch "Sketch50" against normal blind 10 contours A1 A0
extrude "Extrusion47" cut sketch "Sketch50" against normal blind 10 contours L8 L9 A3 A4
extrude "Extrusion48" cut sketch "Sketch50" against normal blind 10 contours A3 L7 L8 A4
extrude "Extrusion49" cut sketch "Sketch50" against normal blind 10 contours A4 A3
sketch "Sketch51" plane through (75.85, 5, 1.5) normal (1, 0, 0) x (0, 0, -1)
  line L0 (-1.5, 0) -> (4.5, 0)
  line L1 (4.5, 0) -> (4.5, -5)
  line L2 (4.5, -5) -> (-1.5, -5)
  line L3 (-1.5, -5) -> (-1.5, 0)
  line L4 (-1.5, 0) -> (4.5, 0)
  line L5 (4.5, 0) -> (4.5, 1)
  line L6 (4.5, 1) -> (-1.5, 1)
  line L7 (-1.5, 1) -> (-1.5, 0)
  point P0 (1.5, -5)
  point P1 (4.5, 0)
  dimension "d128" = 5
  dimension "d129" = 1
  constraints: 16 end point, 4 parallel, 2 horizontal, 2 perpendicular
  measures "d128" distance of L0.end L1.end
  measures "d129" distance of L5.end L4.end
extrude "Extrusion50" add sketch "Sketch51" along normal blind 5 contours L0 L1 L2 L3
extrude "Extrusion51" add sketch "Sketch51" along normal blind 5 contours L7 L6 L5 L0
sketch "Sketch52" plane through (13.859, 5, -1.5) normal (-1, 0, 0) x (0, 0, 1)
  line L0 (-1.5, -5) -> (-1.5, 1) projected
  line L1 (4.5, -5) -> (-1.5, -5) projected
  line L2 (-1.5, 1) -> (4.5, 1)
  line L3 (4.5, 1) -> (4.5, -5)
  line L4 (4.5, -5) -> (-1.5, -5)
  line L5 (-1.5, -5) -> (-1.5, 1)
  point P0 (1.5, -5)
  constraints: 8 end point, 2 parallel, 1 horizontal, 1 perpendicular
extrude "Extrusion52" add sketch "Sketch52" along normal blind 5
sketch "Sketch53" plane through (13.859, 5, -1.5) normal (1, 0, 0) x (0, 0, -1)
  line L0 (-4.5, 1) -> (-4.5, -1.5) projected
  line L1 (1.5, -5) -> (1.5, -2.5) projected
  line L2 (-4.5, 1) -> (1.5, 1)
  line L3 (1.5, 1) -> (1.5, -5)
  line L4 (1.5, -5) -> (-4.5, -5)
  line L5 (-4.5, -5) -> (-4.5, 1)
  point P0 (-1.5, -5)
  constraints: 8 end point, 2 parallel, 1 horizontal, 1 perpendicular
extrude "Extrusion53" add sketch "Sketch53" along normal blind 2
sketch "Sketch54" plane through (75.85, 5, 1.5) normal (-1, 0, 0) x (0, 0, 1)
  line L0 (-4.5, -5) -> (1.5, -5) projected
  line L1 (1.5, 1) -> (-4.5, 1) projected
  line L2 (-4.5, -5) -> (1.5, -5)
  line L3 (1.5, -5) -> (1.5, 1)
  line L4 (1.5, 1) -> (-4.5, 1)
  line L5 (-4.5, 1) -> (-4.5, -5)
  point P0 (-1.5, -5)
  constraints: 8 end point, 2 parallel, 1 horizontal, 1 perpendicular
extrude "Extrusion54" add sketch "Sketch54" along normal blind 2
sketch "Sketch55" plane through (80.85, 5, 1.5) normal (1, 0, 0) x (0, 0, -1)
  circle A0 centre (1.5, -2) radius 1.95
  point P0 (1.5, -5)
  dimension "d140" = 3.9
  constraints: 1 centre point
  measures "d140" diameter of A0
extrude "Extrusion55" cut sketch "Sketch55" against normal blind 6
sketch "Sketch56" plane through (8.859, 5, -1.5) normal (-1, 0, 0) x (0, 0, 1)
  circle A0 centre (1.5, -2) radius 1.95
  point P0 (1.5, -5)
  dimension "d143" = 3.9
  constraints: 1 centre point
  measures "d143" diameter of A0
extrude "Extrusion56" cut sketch "Sketch56" against normal blind 6
fillet "Fillet5" radius 2 4 edges at (12.359, 6, 3) (12.359, 0, 3) (12.359, 6, -3) (12.359, 0, -3)
fillet "Fillet6" radius 2 4 edges at (77.35, 6, 3) (77.35, 6, -3) (77.35, 0, -3) (77.35, 0, 3)
body "Solid1"
